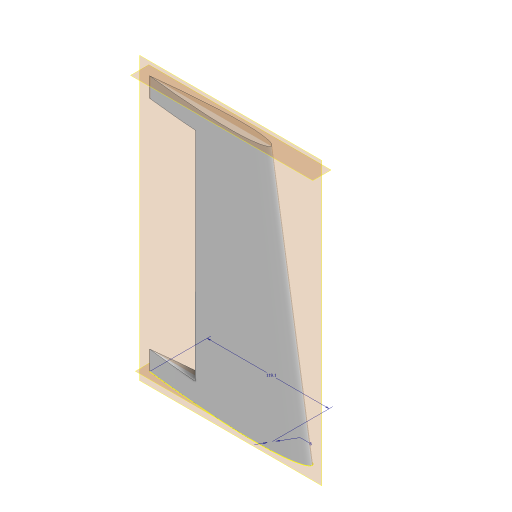
# Autodesk Inventor part: 5P.00.02.01-IB-VTP-Body-Updated
Saved by Autodesk Inventor 2024 (Build 280153000, 153)
## iProperties
Created: 2024-11-08
Part Number: 5P.00.02.01-IB-VTP-Body-Updated
Material: Generic
Document SubType Name: Modeling
Designer: inigo
Density: 1 g/cm^3
Appearance: Default
Author: inigo
Autodesk Inventor part; units mm, degrees
ref_plane "YZ Plane" through (0, 0, 0) normal (1, 0, 0) x (0, 1, 0)
sketch "Sketch1" plane through (0, 0, 0) normal (0, 1, 0) x (-1, 0, 0)
  spline S0 degree 4 poles (118.9, 0) (117.9094, 0.1199) (116.5223, 0.2857) (114.7389, 0.4941) (112.559, 0.743) (110.9735, 0.9211) (109.3882, 1.0958) (107.8029, 1.268) (106.2175, 1.4375) (104.6322, 1.604) (103.0469, 1.768) (101.4615, 1.9292) (99.8762, 2.0878) (98.2909, 2.244) (96.7055, 2.3974) (95.1202, 2.5484) (93.5349, 2.6969) (91.9495, 2.843) (90.3642, 2.9863) (88.7789, 3.1273) (87.1934, 3.2659) (85.6082, 3.4017) (84.0229, 3.5352) (82.4374, 3.666) (80.8522, 3.7941) (79.2669, 3.9198) (77.6814, 4.0426) (76.0961, 4.1626) (74.5109, 4.2801) (72.9254, 4.3944) (71.3402, 4.506) (69.7549, 4.6144) (68.1694, 4.7199) (66.5841, 4.8218) (64.9989, 4.9207) (63.4134, 5.016) (61.8282, 5.1079) (60.2429, 5.1959) (58.6574, 5.2801) (57.0722, 5.3605) (55.4869, 5.4364) (53.9014, 5.5081) (52.3161, 5.5754) (50.7309, 5.6378) (49.1454, 5.6955) (47.5601, 5.7478) (45.9748, 5.7947) (44.3894, 5.8359) (42.8041, 5.8711) (41.2188, 5.9003) (39.6333, 5.9227) (38.048, 5.9381) (36.4627, 5.9461) (34.8773, 5.9467) (33.2919, 5.9387) (31.7066, 5.9222) (30.1211, 5.8965) (28.5358, 5.8605) (26.9504, 5.8146) (25.3649, 5.757) (23.7795, 5.6874) (22.1941, 5.6049) (20.6085, 5.5077) (19.023, 5.3954) (17.4375, 5.2657) (15.8517, 5.1173) (14.266, 4.9472) (12.6798, 4.753) (11.0939, 4.531) (9.5054, 4.2744) (7.9218, 3.9816) (6.3178, 3.6232) (4.7391, 3.2293) (2.9786, 2.5996) (1.6439, 2.136) (-1.1386, 0) (1.6439, -2.136) (2.9786, -2.5996) (4.7391, -3.2293) (6.3178, -3.6232) (7.9218, -3.9816) (9.5054, -4.2744) (11.0939, -4.531) (12.6798, -4.753) (14.266, -4.9472) (15.8517, -5.1173) (17.4375, -5.2657) (19.023, -5.3954) (20.6085, -5.5077) (22.1941, -5.6049) (23.7795, -5.6874) (25.3649, -5.757) (26.9504, -5.8146) (28.5358, -5.8605) (30.1211, -5.8965) (31.7066, -5.9222) (33.2919, -5.9387) (34.8773, -5.9467) (36.4627, -5.9461) (38.048, -5.9381) (39.6333, -5.9227) (41.2188, -5.9003) (42.8041, -5.8711) (44.3894, -5.8359) (45.9748, -5.7947) (47.5601, -5.7478) (49.1454, -5.6955) (50.7309, -5.6378) (52.3161, -5.5754) (53.9014, -5.5081) (55.4869, -5.4364) (57.0722, -5.3605) (58.6574, -5.2801) (60.2429, -5.1959) (61.8282, -5.1079) (63.4134, -5.016) (64.9989, -4.9207) (66.5841, -4.8218) (68.1694, -4.7199) (69.7549, -4.6144) (71.3402, -4.506) (72.9254, -4.3944) (74.5109, -4.2801) (76.0961, -4.1626) (77.6814, -4.0426) (79.2669, -3.9198) (80.8522, -3.7941) (82.4374, -3.666) (84.0229, -3.5352) (85.6082, -3.4017) (87.1934, -3.2659) (88.7789, -3.1273) (90.3642, -2.9863) (91.9495, -2.843) (93.5349, -2.6969) (95.1202, -2.5484) (96.7055, -2.3974) (98.2909, -2.244) (99.8762, -2.0878) (101.4615, -1.9292) (103.0469, -1.768) (104.6322, -1.604) (106.2175, -1.4375) (107.8029, -1.268) (109.3882, -1.0958) (110.9735, -0.9211) (112.559, -0.743) (114.7389, -0.4941) (116.5223, -0.2857) (117.9094, -0.1199) (118.9, 0) knots 0 0 0 0 0 0.016619 0.023265 0.029911 0.036556 0.0432 0.049844 0.056487 0.06313 0.069772 0.076413 0.083054 0.089694 0.096334 0.102973 0.109612 0.11625 0.122888 0.129526 0.136163 0.142799 0.149435 0.156071 0.162706 0.169341 0.175975 0.182609 0.189242 0.195875 0.202508 0.20914 0.215771 0.222403 0.229034 0.235664 0.242294 0.248923 0.255552 0.262181 0.268809 0.275437 0.282064 0.288691 0.295318 0.301944 0.30857 0.315195 0.321821 0.328446 0.33507 0.341695 0.34832 0.354944 0.361569 0.368194 0.374819 0.381445 0.388072 0.394699 0.401328 0.407958 0.41459 0.421225 0.427863 0.434505 0.441152 0.447806 0.45447 0.461148 0.467846 0.474578 0.481378 0.488582 0.496181 0.503819 0.511418 0.518622 0.525422 0.532154 0.538852 0.54553 0.552194 0.558848 0.565495 0.572137 0.578775 0.58541 0.592042 0.598672 0.605301 0.611928 0.618555 0.625181 0.631806 0.638431 0.645056 0.65168 0.658305 0.66493 0.671554 0.678179 0.684805 0.69143 0.698056 0.704682 0.711309 0.717936 0.724563 0.731191 0.737819 0.744448 0.751077 0.757706 0.764336 0.770966 0.777597 0.784229 0.79086 0.797492 0.804125 0.810758 0.817391 0.824025 0.830659 0.837294 0.843929 0.850565 0.857201 0.863837 0.870474 0.877112 0.88375 0.890388 0.897027 0.903666 0.910306 0.916946 0.923587 0.930228 0.93687 0.943513 0.950156 0.9568 0.963444 0.970089 0.976735 0.983381 1 1 1 1 1
  point P0 (0, 0)
  point P1 (115.7293, 0.3775)
  point P2 (114.144, 0.5614)
  point P3 (112.5587, 0.7424)
  point P4 (110.9733, 0.9204)
  point P5 (109.388, 1.0953)
  point P6 (107.8027, 1.2675)
  point P7 (106.2173, 1.4369)
  point P8 (104.632, 1.6035)
  point P9 (103.0467, 1.7674)
  point P10 (101.4613, 1.9287)
  point P11 (99.876, 2.0873)
  point P12 (98.2907, 2.2434)
  point P13 (96.7053, 2.3969)
  point P14 (95.12, 2.5479)
  point P15 (93.5347, 2.6964)
  point P16 (91.9493, 2.8424)
  point P17 (90.364, 2.9858)
  point P18 (88.7787, 3.1268)
  point P19 (87.1933, 3.2654)
  point P20 (85.608, 3.4013)
  point P21 (84.0227, 3.5347)
  point P22 (82.4373, 3.6654)
  point P23 (80.852, 3.7936)
  point P24 (79.2667, 3.9192)
  point P25 (77.6813, 4.042)
  point P26 (76.096, 4.1621)
  point P27 (74.5107, 4.2794)
  point P28 (72.9253, 4.3938)
  point P29 (71.34, 4.5054)
  point P30 (69.7547, 4.6138)
  point P31 (68.1693, 4.7191)
  point P32 (66.584, 4.8212)
  point P33 (64.9987, 4.92)
  point P34 (63.4133, 5.0153)
  point P35 (61.828, 5.1071)
  point P36 (60.2427, 5.1951)
  point P37 (58.6573, 5.2793)
  point P38 (57.072, 5.3595)
  point P39 (55.4867, 5.4355)
  point P40 (53.9013, 5.5072)
  point P41 (52.316, 5.5744)
  point P42 (50.7307, 5.6368)
  point P43 (49.1453, 5.6944)
  point P44 (47.56, 5.7467)
  point P45 (45.9747, 5.7935)
  point P46 (44.3893, 5.8347)
  point P47 (42.804, 5.8699)
  point P48 (41.2187, 5.8989)
  point P49 (39.6333, 5.9212)
  point P50 (38.048, 5.9366)
  point P51 (36.4627, 5.9445)
  point P52 (34.8773, 5.9449)
  point P53 (33.292, 5.9369)
  point P54 (31.7067, 5.9203)
  point P55 (30.1213, 5.8943)
  point P56 (28.536, 5.8584)
  point P57 (26.9507, 5.8122)
  point P58 (25.3653, 5.7545)
  point P59 (23.78, 5.6847)
  point P60 (22.1947, 5.6019)
  point P61 (20.6093, 5.5046)
  point P62 (19.024, 5.3919)
  point P63 (17.4387, 5.2619)
  point P64 (15.8533, 5.1129)
  point P65 (14.268, 4.9424)
  point P66 (12.6827, 4.7476)
  point P67 (11.0973, 4.5244)
  point P68 (9.512, 4.2678)
  point P69 (7.9267, 3.97)
  point P70 (6.3413, 3.6198)
  point P71 (4.756, 3.1982)
  point P72 (3.1707, 2.668)
  point P73 (1.5853, 1.9346)
  point P74 (0, 0)
  point P75 (1.5853, -1.9346)
  point P76 (3.1707, -2.668)
  point P77 (4.756, -3.1982)
  point P78 (6.3413, -3.6198)
  point P79 (7.9267, -3.97)
  point P80 (9.512, -4.2678)
  point P81 (11.0973, -4.5244)
  point P82 (12.6827, -4.7476)
  point P83 (14.268, -4.9424)
  point P84 (15.8533, -5.1129)
  point P85 (17.4387, -5.2619)
  point P86 (19.024, -5.3919)
  point P87 (20.6093, -5.5046)
  point P88 (22.1947, -5.6019)
  point P89 (23.78, -5.6847)
  point P90 (25.3653, -5.7545)
  point P91 (26.9507, -5.8122)
  point P92 (28.536, -5.8584)
  point P93 (30.1213, -5.8943)
  point P94 (31.7067, -5.9203)
  point P95 (33.292, -5.9369)
  point P96 (34.8773, -5.9449)
  point P97 (36.4627, -5.9445)
  point P98 (38.048, -5.9366)
  point P99 (39.6333, -5.9212)
  point P100 (41.2187, -5.8989)
  point P101 (42.804, -5.8699)
  point P102 (44.3893, -5.8347)
  point P103 (45.9747, -5.7935)
  point P104 (47.56, -5.7467)
  point P105 (49.1453, -5.6944)
  point P106 (50.7307, -5.6368)
  point P107 (52.316, -5.5744)
  point P108 (53.9013, -5.5072)
  point P109 (55.4867, -5.4355)
  point P110 (57.072, -5.3595)
  point P111 (58.6573, -5.2793)
  point P112 (60.2427, -5.1951)
  point P113 (61.828, -5.1071)
  point P114 (63.4133, -5.0153)
  point P115 (64.9987, -4.92)
  point P116 (66.584, -4.8212)
  point P117 (68.1693, -4.7191)
  point P118 (69.7547, -4.6138)
  point P119 (71.34, -4.5054)
  point P120 (72.9253, -4.3938)
  point P121 (74.5107, -4.2794)
  point P122 (76.096, -4.1621)
  point P123 (77.6813, -4.042)
  point P124 (79.2667, -3.9192)
  point P125 (80.852, -3.7936)
  point P126 (82.4373, -3.6654)
  point P127 (84.0227, -3.5347)
  point P128 (85.608, -3.4013)
  point P129 (87.1933, -3.2654)
  point P130 (88.7787, -3.1268)
  point P131 (90.364, -2.9858)
  point P132 (91.9493, -2.8424)
  point P133 (93.5347, -2.6964)
  point P134 (95.12, -2.5479)
  point P135 (96.7053, -2.3969)
  point P136 (98.2907, -2.2434)
  point P137 (99.876, -2.0873)
  point P138 (101.4613, -1.9287)
  point P139 (103.0467, -1.7674)
  point P140 (104.632, -1.6035)
  point P141 (106.2173, -1.4369)
  point P142 (107.8027, -1.2675)
  point P143 (109.388, -1.0953)
  point P144 (110.9733, -0.9204)
  point P145 (112.5587, -0.7424)
  point P146 (114.144, -0.5614)
  point P147 (115.7293, -0.3775)
  point P148 (117.3147, -0.1904)
  constraints: 151 other
ref_plane "Work Plane1" through (0, -250, 0) normal (0, 1, 0) x (-1, 0, 0)
sketch "Sketch2" plane through (0, -250, 0) normal (0, 1, 0) x (-1, 0, 0)
  spline S0 degree 4 poles (118.95, 0) (117.6287, 0.1599) (115.7784, 0.3811) (113.3995, 0.6591) (110.4917, 0.9911) (108.3769, 1.2286) (106.2623, 1.4617) (104.1477, 1.6914) (102.0329, 1.9175) (99.9183, 2.1395) (97.8037, 2.3584) (95.6889, 2.5733) (93.5742, 2.7849) (91.4596, 2.9932) (89.3448, 3.1979) (87.2302, 3.3993) (85.1156, 3.5974) (83.0008, 3.7923) (80.8862, 3.9834) (78.7716, 4.1716) (76.6568, 4.3564) (74.5422, 4.5375) (72.4276, 4.7156) (70.3128, 4.89) (68.1982, 5.061) (66.0836, 5.2285) (63.9688, 5.3924) (61.8542, 5.5525) (59.7396, 5.7092) (57.6248, 5.8616) (55.5102, 6.0106) (53.3956, 6.1551) (51.2808, 6.2958) (49.1662, 6.4317) (47.0516, 6.5637) (44.9368, 6.6908) (42.8222, 6.8134) (40.7076, 6.9307) (38.5928, 7.043) (36.4782, 7.1503) (34.3636, 7.2515) (32.2488, 7.3473) (30.1342, 7.437) (28.0196, 7.5202) (25.9048, 7.5971) (23.7902, 7.667) (21.6756, 7.7295) (19.5607, 7.7845) (17.4461, 7.8314) (15.3315, 7.8703) (13.2167, 7.9002) (11.1021, 7.9208) (8.9874, 7.9314) (6.8726, 7.9322) (4.7579, 7.9216) (2.6433, 7.8996) (0.5284, 7.8653) (-1.5863, 7.8173) (-3.701, 7.7561) (-5.8159, 7.6792) (-7.9306, 7.5864) (-10.0454, 7.4763) (-12.1604, 7.3467) (-14.2753, 7.1969) (-16.3902, 7.0239) (-18.5056, 6.8259) (-20.6207, 6.5991) (-22.7365, 6.3399) (-24.8519, 6.0438) (-26.9708, 5.7017) (-29.0832, 5.311) (-31.2227, 4.833) (-33.3285, 4.3076) (-35.6769, 3.4676) (-37.4572, 2.8492) (-41.1688, 0) (-37.4572, -2.8492) (-35.6769, -3.4676) (-33.3285, -4.3076) (-31.2227, -4.833) (-29.0832, -5.311) (-26.9708, -5.7017) (-24.8519, -6.0438) (-22.7365, -6.3399) (-20.6207, -6.5991) (-18.5056, -6.8259) (-16.3902, -7.0239) (-14.2753, -7.1969) (-12.1604, -7.3467) (-10.0454, -7.4763) (-7.9306, -7.5864) (-5.8159, -7.6792) (-3.701, -7.7561) (-1.5863, -7.8173) (0.5284, -7.8653) (2.6433, -7.8996) (4.7579, -7.9216) (6.8726, -7.9322) (8.9874, -7.9314) (11.1021, -7.9208) (13.2167, -7.9002) (15.3315, -7.8703) (17.4461, -7.8314) (19.5607, -7.7845) (21.6756, -7.7295) (23.7902, -7.667) (25.9048, -7.5971) (28.0196, -7.5202) (30.1342, -7.437) (32.2488, -7.3473) (34.3636, -7.2515) (36.4782, -7.1503) (38.5928, -7.043) (40.7076, -6.9307) (42.8222, -6.8134) (44.9368, -6.6908) (47.0516, -6.5637) (49.1662, -6.4317) (51.2808, -6.2958) (53.3956, -6.1551) (55.5102, -6.0106) (57.6248, -5.8616) (59.7396, -5.7092) (61.8542, -5.5525) (63.9688, -5.3924) (66.0836, -5.2285) (68.1982, -5.061) (70.3128, -4.89) (72.4276, -4.7156) (74.5422, -4.5375) (76.6568, -4.3564) (78.7716, -4.1716) (80.8862, -3.9834) (83.0008, -3.7923) (85.1156, -3.5974) (87.2302, -3.3993) (89.3448, -3.1979) (91.4596, -2.9932) (93.5742, -2.7849) (95.6889, -2.5733) (97.8037, -2.3584) (99.9183, -2.1395) (102.0329, -1.9175) (104.1477, -1.6914) (106.2623, -1.4617) (108.3769, -1.2286) (110.4917, -0.9911) (113.3995, -0.6591) (115.7784, -0.3811) (117.6287, -0.1599) (118.95, 0) knots 0 0 0 0 0 0.016619 0.023265 0.029911 0.036556 0.0432 0.049844 0.056487 0.06313 0.069772 0.076413 0.083054 0.089694 0.096334 0.102973 0.109612 0.11625 0.122888 0.129526 0.136163 0.142799 0.149435 0.156071 0.162706 0.169341 0.175975 0.182609 0.189242 0.195875 0.202508 0.20914 0.215771 0.222403 0.229034 0.235664 0.242294 0.248923 0.255552 0.262181 0.268809 0.275437 0.282064 0.288691 0.295318 0.301944 0.30857 0.315195 0.321821 0.328446 0.33507 0.341695 0.34832 0.354944 0.361569 0.368194 0.374819 0.381445 0.388072 0.394699 0.401328 0.407958 0.41459 0.421225 0.427863 0.434505 0.441152 0.447806 0.45447 0.461148 0.467846 0.474578 0.481378 0.488582 0.496181 0.503819 0.511418 0.518622 0.525422 0.532154 0.538852 0.54553 0.552194 0.558848 0.565495 0.572137 0.578775 0.58541 0.592042 0.598672 0.605301 0.611928 0.618555 0.625181 0.631806 0.638431 0.645056 0.65168 0.658305 0.66493 0.671554 0.678179 0.684805 0.69143 0.698056 0.704682 0.711309 0.717936 0.724563 0.731191 0.737819 0.744448 0.751077 0.757706 0.764336 0.770966 0.777597 0.784229 0.79086 0.797492 0.804125 0.810758 0.817391 0.824025 0.830659 0.837294 0.843929 0.850565 0.857201 0.863837 0.870474 0.877112 0.88375 0.890388 0.897027 0.903666 0.910306 0.916946 0.923587 0.930228 0.93687 0.943513 0.950156 0.9568 0.963444 0.970089 0.976735 0.983381 1 1 1 1 1
  point P0 (0, 0)
  point P1 (114.7206, 0.5036)
  point P2 (112.606, 0.7489)
  point P3 (110.4914, 0.9903)
  point P4 (108.3766, 1.2277)
  point P5 (106.262, 1.461)
  point P6 (104.1474, 1.6907)
  point P7 (102.0326, 1.9167)
  point P8 (99.918, 2.1389)
  point P9 (97.8034, 2.3576)
  point P10 (95.6886, 2.5727)
  point P11 (93.574, 2.7842)
  point P12 (91.4594, 2.9925)
  point P13 (89.3446, 3.1972)
  point P14 (87.23, 3.3986)
  point P15 (85.1154, 3.5967)
  point P16 (83.0006, 3.7915)
  point P17 (80.886, 3.9828)
  point P18 (78.7714, 4.1709)
  point P19 (76.6566, 4.3556)
  point P20 (74.542, 4.5369)
  point P21 (72.4274, 4.7149)
  point P22 (70.3126, 4.8893)
  point P23 (68.198, 5.0603)
  point P24 (66.0834, 5.2278)
  point P25 (63.9686, 5.3916)
  point P26 (61.854, 5.5518)
  point P27 (59.7394, 5.7083)
  point P28 (57.6246, 5.8609)
  point P29 (55.51, 6.0097)
  point P30 (53.3954, 6.1543)
  point P31 (51.2806, 6.2948)
  point P32 (49.166, 6.4309)
  point P33 (47.0514, 6.5627)
  point P34 (44.9366, 6.6899)
  point P35 (42.822, 6.8123)
  point P36 (40.7074, 6.9297)
  point P37 (38.5926, 7.042)
  point P38 (36.478, 7.1491)
  point P39 (34.3634, 7.2504)
  point P40 (32.2486, 7.346)
  point P41 (30.134, 7.4356)
  point P42 (28.0194, 7.5189)
  point P43 (25.9046, 7.5957)
  point P44 (23.79, 7.6655)
  point P45 (21.6754, 7.7279)
  point P46 (19.5606, 7.7828)
  point P47 (17.446, 7.8298)
  point P48 (15.3314, 7.8685)
  point P49 (13.2166, 7.8983)
  point P50 (11.102, 7.9187)
  point P51 (8.9874, 7.9294)
  point P52 (6.8726, 7.9298)
  point P53 (4.758, 7.9192)
  point P54 (2.6434, 7.897)
  point P55 (0.5286, 7.8624)
  point P56 (-1.586, 7.8145)
  point P57 (-3.7006, 7.7528)
  point P58 (-5.8154, 7.6759)
  point P59 (-7.93, 7.5828)
  point P60 (-10.0446, 7.4723)
  point P61 (-12.1594, 7.3425)
  point P62 (-14.274, 7.1922)
  point P63 (-16.3886, 7.0188)
  point P64 (-18.5034, 6.8201)
  point P65 (-20.618, 6.5927)
  point P66 (-22.7326, 6.3327)
  point P67 (-24.8474, 6.035)
  point P68 (-26.962, 5.6928)
  point P69 (-29.0766, 5.2955)
  point P70 (-31.1914, 4.8284)
  point P71 (-33.306, 4.266)
  point P72 (-35.4206, 3.5588)
  point P73 (-37.5354, 2.5806)
  point P74 (-39.65, 0)
  point P75 (-37.5354, -2.5806)
  point P76 (-35.4206, -3.5588)
  point P77 (-33.306, -4.266)
  point P78 (-31.1914, -4.8284)
  point P79 (-29.0766, -5.2955)
  point P80 (-26.962, -5.6928)
  point P81 (-24.8474, -6.035)
  point P82 (-22.7326, -6.3327)
  point P83 (-20.618, -6.5927)
  point P84 (-18.5034, -6.8201)
  point P85 (-16.3886, -7.0188)
  point P86 (-14.274, -7.1922)
  point P87 (-12.1594, -7.3425)
  point P88 (-10.0446, -7.4723)
  point P89 (-7.93, -7.5828)
  point P90 (-5.8154, -7.6759)
  point P91 (-3.7006, -7.7528)
  point P92 (-1.586, -7.8145)
  point P93 (0.5286, -7.8624)
  point P94 (2.6434, -7.897)
  point P95 (4.758, -7.9192)
  point P96 (6.8726, -7.9298)
  point P97 (8.9874, -7.9294)
  point P98 (11.102, -7.9187)
  point P99 (13.2166, -7.8983)
  point P100 (15.3314, -7.8685)
  point P101 (17.446, -7.8298)
  point P102 (19.5606, -7.7828)
  point P103 (21.6754, -7.7279)
  point P104 (23.79, -7.6655)
  point P105 (25.9046, -7.5957)
  point P106 (28.0194, -7.5189)
  point P107 (30.134, -7.4356)
  point P108 (32.2486, -7.346)
  point P109 (34.3634, -7.2504)
  point P110 (36.478, -7.1491)
  point P111 (38.5926, -7.042)
  point P112 (40.7074, -6.9297)
  point P113 (42.822, -6.8123)
  point P114 (44.9366, -6.6899)
  point P115 (47.0514, -6.5627)
  point P116 (49.166, -6.4309)
  point P117 (51.2806, -6.2948)
  point P118 (53.3954, -6.1543)
  point P119 (55.51, -6.0097)
  point P120 (57.6246, -5.8609)
  point P121 (59.7394, -5.7083)
  point P122 (61.854, -5.5518)
  point P123 (63.9686, -5.3916)
  point P124 (66.0834, -5.2278)
  point P125 (68.198, -5.0603)
  point P126 (70.3126, -4.8893)
  point P127 (72.4274, -4.7149)
  point P128 (74.542, -4.5369)
  point P129 (76.6566, -4.3556)
  point P130 (78.7714, -4.1709)
  point P131 (80.886, -3.9828)
  point P132 (83.0006, -3.7915)
  point P133 (85.1154, -3.5967)
  point P134 (87.23, -3.3986)
  point P135 (89.3446, -3.1972)
  point P136 (91.4594, -2.9925)
  point P137 (93.574, -2.7842)
  point P138 (95.6886, -2.5727)
  point P139 (97.8034, -2.3576)
  point P140 (99.918, -2.1389)
  point P141 (102.0326, -1.9167)
  point P142 (104.1474, -1.6907)
  point P143 (106.262, -1.461)
  point P144 (108.3766, -1.2277)
  point P145 (110.4914, -0.9903)
  point P146 (112.606, -0.7489)
  point P147 (114.7206, -0.5036)
  point P148 (116.8354, -0.2539)
  constraints: 151 other
loft "Loft1" add profiles "Sketch2", "Sketch1"
sketch "Sketch3" plane through (0, 0, 0) normal (0, 0, 1) x (1, 0, 0)
  line L0 (-118.95, -250) -> (-118.9, 0) projected
  line L1 (-118.9038, -18.985) -> (-69.4038, -18.985)
  line L2 (-69.4038, -18.985) -> (-69.4038, -231.015)
  line L3 (-69.4038, -231.015) -> (-118.9038, -231.015)
  line L4 (-150.9855, 0) -> (73.1945, 0) projected
  line L5 (-118.9038, -18.985) -> (-182.772, -18.985)
  line L6 (-182.772, -18.985) -> (-182.772, -231.015)
  line L7 (-182.772, -231.015) -> (-118.9038, -231.015)
  point P0 (0, 0)
  dimension "d5" = 49.5
  dimension "d6" = 212.03
  dimension "d7" = 18.985
  constraints: 12 end point, 2 horizontal, 2 parallel, 2 perpendicular, 1 point on line
  measures "d5" distance of L1.start L1.end
  measures "d6" distance of L1.end L2.end
  measures "d7" distance between parallel lines of L4 L1
split body "Split1" sketch "Sketch3" result two bodies curves L1 L2 L3 L7 L6 L5 first body at (-62.3919, -170.7557, -4.9005)
sketch "Sketch4" plane through (0, -250, 0) normal (0, 1, 0) x (-1, 0, 0)
  circle A0 centre (-0.15, 0) radius 3
  point P0 (0, 0)
  dimension "d8" = 6
  dimension "d9" = 119.1
  constraints: 1 centre point, 1 other
  measures "d8" diameter of A0
  measures "d9" distance of point (118.95, 0) A0.centre
equation "\"d5\" = rudWidth"
equation "\"d6\" = rudHeight"
equation "\"d7\" = overhang"
equation "\"rudHeight\" = 212.03"
equation "\"rudWidth\" = 49.5"
equation "\"overhang\" = 18.985"
body "Solid2"
body "Solid3"
